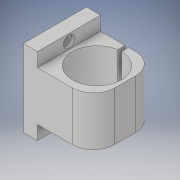
# Autodesk Inventor part: Cleaning Bottle Holder
Saved by Autodesk Inventor 2019 (Build 230136000, 136)
## iProperties
Created: 2019-01-17
Part Number: Cleaning Bottle Holder
Material: Generic
Document SubType Name: Modeling
Designer: dewanlab
Density: 1 g/cm^3
Appearance: Default
Author: dewanlab
Autodesk Inventor part; units mm, degrees
ref_plane "YZ Plane" through (0, 0, 0) normal (1, 0, 0) x (0, 1, 0)
ref_plane "XZ Plane" through (0, 0, 0) normal (0, 1, 0) x (-1, 0, 0)
ref_plane "XY Plane" through (0, 0, 0) normal (0, 0, 1) x (1, 0, 0)
sketch "Sketch1" plane through (0, 0, 0) normal (1, 0, 0) x (0, 1, 0)
  line L0 (112.7241, 89.8734) -> (-26.9759, 89.8734)
  line L1 (-26.9759, 89.8734) -> (-26.9759, -24.4266)
  line L2 (-26.9759, -24.4266) -> (112.7241, -24.4266)
  line L3 (112.7241, -24.4266) -> (112.7241, 89.8734)
  point P0 (0, 0)
  dimension "d0" = 114.3
  dimension "d1" = 139.7
  constraints: 8 end point, 2 parallel, 1 horizontal, 1 perpendicular
  measures "d0" distance between parallel lines of L2 L0
  measures "d1" distance between parallel lines of L1 L3
extrude "Extrusion1" add sketch "Sketch1" along normal blind 127
sketch "Sketch2" plane through (0, 112.7241, 89.8734) normal (0, 1, 0) x (1, 0, 0)
  line L0 (0, 0) -> (127, 0) projected
  line L1 (0, 114.3) -> (127, 114.3) projected
  line L2 (25.4, 0) -> (127, 0)
  line L3 (127, 0) -> (127, 114.3)
  line L4 (127, 114.3) -> (25.4, 114.3)
  line L5 (25.4, 114.3) -> (25.4, 0)
  line L6 (0, 114.3) -> (0, 0) projected
  point P0 (0, 89.8734)
  dimension "d4" = 25.4
  constraints: 8 end point, 2 parallel, 1 horizontal, 1 perpendicular, 1 point on line
  measures "d4" distance between parallel lines of L5 L6
extrude "Extrusion2" cut sketch "Sketch2" against normal blind 25.4 contours L5 L1 L3 L0
sketch "Sketch4" plane through (0, 87.3241, 89.8734) normal (0, 1, 0) x (1, 0, 0)
  line L0 (38.1, 127) -> (38.1, 0) projected
  circle A0 centre (76.2, 57.15) radius 44.45
  line L1 (127, 114.3) -> (127, 0) projected
  line L2 (127, 0) -> (25.4, 0) projected
  point P0 (0, 89.8734)
  dimension "d15" = 50.8
  dimension "d16" = 57.15
  dimension "d54" = 88.9
  constraints: 1 centre point
  measures "d15" distance from line of L1 A0.centre
  measures "d16" distance from line of L2 A0.centre
  measures "d54" diameter of A0
extrude "Extrusion4" cut sketch "Sketch4" against normal blind 63.5
fillet "Fillet3" radius 38.1 1 edges at (127, 30.1741, 89.8734)
fillet "Fillet4" radius 38.1 1 edges at (127, 30.1741, -24.4266)
sketch "Sketch9" plane through (25.4, 112.7241, 89.8734) normal (1, 0, 0) x (0, 0, -1)
  line L0 (0, 0) -> (114.3, 0) projected
  line L1 (0, -25.4) -> (0, 0) projected
  point P0 (89.8734, -112.7241)
  point P1 (57.15, -12.7)
  dimension "d30" = 12.7
  dimension "d31" = 57.15
  measures "d30" distance from line of point (57.15, -12.7) L0
  measures "d31" distance from line of L1 point (57.15, -12.7)
hole "Hole1" at (25.4, 100.0241, 32.7234) direction (-1, 0, 0) diameter 8.4328 end through all counterbore diameter 20.6502 counterbore depth 5.969 clearance for "Hex Head Bolt" size "5/16" standard "Ansi Unified Screw Threads"
sketch "Sketch10" plane through (0, -26.9759, -24.4266) normal (0, -1, 0) x (1, 0, 0)
  line L0 (0, 114.3) -> (88.9, 114.3) projected
  line L1 (25.4, 114.3) -> (127, 114.3)
  line L2 (127, 114.3) -> (127, 0)
  line L3 (127, 0) -> (25.4, 0)
  line L4 (25.4, 0) -> (25.4, 114.3)
  line L5 (0, 114.3) -> (0, 0) projected
  point P0 (0, 24.4266)
  dimension "d39" = 25.4
  dimension "d42" = 114.3
  dimension "d60" = 101.6
  constraints: 8 end point, 2 parallel, 1 horizontal, 1 perpendicular, 1 point on line
  measures "d39" distance between parallel lines of L5 L4
  measures "d42" distance between parallel lines of L3 L1
  measures "d60" distance between parallel lines of L2 L4
extrude "Extrusion6" cut sketch "Sketch10" against normal blind 25.4
sketch "Sketch11" plane through (25.4, -26.9759, 89.8734) normal (1, 0, 0) x (0, 0, -1)
  line L0 (114.3, 0) -> (0, 0) projected
  line L1 (114.3, 25.4) -> (114.3, 0) projected
  point P0 (89.8734, 26.9759)
  point P1 (57.15, 12.7)
  dimension "d43" = 12.7
  dimension "d44" = 57.15
  measures "d43" distance from line of L0 point (57.15, 12.7)
  measures "d44" distance from line of L1 point (57.15, 12.7)
hole "Hole2" at (25.4, -14.2759, 32.7234) direction (-1, 0, 0) diameter 8.4328 end through all counterbore diameter 20.6502 counterbore depth 5.969 clearance for "Hex Head Bolt" size "5/16" standard "Ansi Unified Screw Threads"
sketch "Sketch15" plane through (0, -26.9759, -24.4266) normal (0, 0, -1) x (-1, 0, 0)
  line L0 (-25.4, 114.3) -> (-88.9, 114.3) projected
  line L1 (-76.2, 114.3) -> (-69.85, 114.3)
  line L2 (-69.85, 114.3) -> (-69.85, 50.8)
  line L3 (-69.85, 50.8) -> (-76.2, 50.8)
  line L4 (-76.2, 50.8) -> (-76.2, 114.3)
  line L5 (-127, 114.3) -> (-127, 0) projected
  point P0 (0, 26.9759)
  point P1 (-127, 25.4)
  dimension "d55" = 6.35
  dimension "d56" = 50.8
  dimension "d57" = 63.5
  constraints: 8 end point, 2 parallel, 1 horizontal, 1 perpendicular, 1 point on line
  measures "d55" distance between parallel lines of L2 L4
  measures "d56" distance between parallel lines of L5 L4
  measures "d57" distance from line of L2.end L0
extrude "Extrusion8" cut sketch "Sketch15" against normal blind 25.4
body "Solid1"
